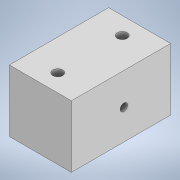
# Autodesk Inventor part: Base Idler Izq
Saved by Autodesk Inventor 2021 (Build 250183000, 183)
## iProperties
Created: 2023-01-27
Part Number: Base Idler Izq
Material: Genérico
Document SubType Name: Modeling
Designer: Diego.labarca
Density: 1 g/cm^3
Appearance: Valor por defecto
Author: Diego.labarca
Autodesk Inventor part; units mm, degrees
ref_plane "YZ Plane" through (0, 0, 0) normal (1, 0, 0) x (0, 1, 0)
ref_plane "XZ Plane" through (0, 0, 0) normal (0, 1, 0) x (-1, 0, 0)
ref_plane "XY Plane" through (0, 0, 0) normal (0, 0, 1) x (1, 0, 0)
sketch "Boceto1" plane through (0, 0, 0) normal (0, 1, 0) x (-1, 0, 0)
  line L0 (12.5, 20) -> (-12.5, 20)
  line L1 (-12.5, 20) -> (-12.5, -20)
  line L2 (-12.5, -20) -> (12.5, -20)
  line L3 (12.5, -20) -> (12.5, 20)
  line L4 (0, -3.0912) -> (0, 0)
  line L5 (0, 0) -> (2.0406, 0)
  circle A0 centre (0, 13) radius 2
  circle A1 centre (0, -13) radius 2
  dimension "d0" = 25
  dimension "d1" = 40
  dimension "d4" = 4
  dimension "d5" = 4
  dimension "d6" = 7
  dimension "d7" = 7
  constraints: 12 end point, 2 centre point, 2 parallel, 2 perpendicular, 1 horizontal, 1 point on line, 1 vertical, 2 other
  measures "d0" distance of L2.end L1.end
  measures "d1" distance of L1.end L0.end
  measures "d4" diameter of A0
  measures "d5" diameter of A1
  measures "d6" distance from line of L0 A0.centre
  measures "d7" distance from line of A1.centre L2
extrude "Extrusión1" add sketch "Boceto1" along normal blind 5
sketch "Boceto2" plane through (0, 0, 0) normal (0, -1, 0) x (1, 0, 0)
  line L0 (12.5, 20) -> (12.5, -20) projected
  line L1 (12.5, 20) -> (7.5, 20)
  line L2 (7.5, 20) -> (7.5, -20)
  line L3 (7.5, -20) -> (12.5, -20)
  line L4 (12.5, -20) -> (12.5, 20)
  line L5 (-12.5, -20) -> (-12.5, 20) projected
  line L6 (-12.5, 20) -> (12.5, 20) projected
  line L7 (-12.5, -20) -> (-7.5, -20)
  line L8 (-7.5, -20) -> (-7.5, 20)
  line L9 (-7.5, 20) -> (-12.5, 20)
  line L10 (-12.5, 20) -> (-12.5, -20)
  point P0 (0, 0)
  dimension "d8" = 5
  dimension "d9" = 5
  constraints: 16 end point, 4 parallel, 2 horizontal, 2 perpendicular, 1 point on line
  measures "d8" distance between parallel lines of L0 L2
  measures "d9" distance between parallel lines of L8 L5
extrude "Extrusión2" add sketch "Boceto2" along normal blind 20
sketch "Boceto3" plane through (-7.5, 0, 20) normal (1, 0, 0) x (0, 0, -1)
  line L0 (0, 0) -> (0, -20) projected
  line L1 (40, -20) -> (40, 5) projected
  line L2 (0, -20) -> (40, -20)
  line L3 (40, -20) -> (40, -16)
  line L4 (40, -16) -> (0, -16)
  line L5 (0, -16) -> (0, -20)
  point P0 (20, 0)
  point P1 (0, -16)
  dimension "d12" = 4
  constraints: 8 end point, 2 parallel, 1 horizontal, 1 perpendicular, 1 point on line
  measures "d12" distance between parallel lines of L2 L4
extrude "Extrusión3" add sketch "Boceto3" along normal up to surface (15 mm away)
sketch "Boceto4" plane through (12.5, 5, 20) normal (1, 0, 0) x (0, 0, -1)
  circle A0 centre (21.15, -12.85) radius 1.5
  line L0 (0, 0) -> (0, -25) projected
  line L1 (0, 0) -> (40, 0) projected
  point P0 (20, -5)
  dimension "d15" = 21.15
  dimension "d16" = 12.85
  dimension "d19" = 3
  constraints: 1 centre point
  measures "d15" distance from line of L0 A0.centre
  measures "d16" distance from line of L1 A0.centre
  measures "d19" diameter of A0
extrude "Extrusión4" cut sketch "Boceto4" against normal up to surface (5 mm away)
sketch "Boceto5" plane through (-12.5, 5, -20) normal (-1, 0, 0) x (0, 0, 1)
  circle A0 centre (18.85, -12.85) radius 1.5 projected
  point P0 (20, -5)
hole "Agujero1" at (-12.5, -7.85, -1.15) direction (1, 0, 0) diameter 4 depth 5
sketch "Boceto6" plane through (-12.5, 5, 20) normal (0, 0, 1) x (1, 0, 0)
  line L0 (5, -5) -> (5, -21) projected
  line L1 (5, -5) -> (20, -5) projected
  line L2 (20, -5) -> (20, -21) projected
  line L3 (5, -21) -> (20, -21) projected
  line L4 (25, -25) -> (0, -25) projected
  line L5 (25, 0) -> (25, -25) projected
  line L6 (0, 0) -> (25, 0) projected
  line L7 (0, -25) -> (0, 0) projected
  point P0 (12.5, -5)
extrude "Extrusión5" add sketch "Boceto6" against normal blind 5 contours L1 L2 L3 L0
sketch "Boceto8" plane through (0, -20, 0) normal (0, -1, 0) x (1, 0, 0)
  circle A0 centre (0, 13) radius 2 projected
  circle A1 centre (0, -13) radius 2 projected
  circle A2 centre (0, 13) radius 2.5
  circle A3 centre (0, -13) radius 2.5
  point P0 (0, 0)
  dimension "d31" = 5
  dimension "d32" = 5
  constraints: 2 centre point, 2 coincident
  measures "d31" diameter of A2
  measures "d32" diameter of A3
extrude "Extrusión7" cut sketch "Boceto8" against normal up to surface (4 mm away) contours A0 | A1 | A2 | A3
equation "\"d5\" = d4"
equation "\"d7\" = d6"
equation "\"d9\" = d8"
